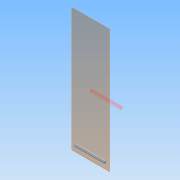
# Autodesk Inventor part: TopBottomBorder
Saved by Autodesk Inventor 2013 (Build 170138000, 138)
## iProperties
Created: 2018-07-18
Part Number: TopBottomBorder
Material: Generic
Document SubType Name: Modeling
Designer: Jeff Vyduna
Density: 1 g/cm^3
Author: Jeff Vyduna
Autodesk Inventor part; units mm, degrees
ref_plane "YZ Plane" through (0, 0, 0) normal (1, 0, 0) x (0, 1, 0)
ref_plane "XZ Plane" through (0, 0, 0) normal (0, 1, 0) x (-1, 0, 0)
ref_plane "XY Plane" through (0, 0, 0) normal (0, 0, 1) x (1, 0, 0)
ref_plane "Work Plane1" through (0, 0, 0) normal (0, 0, 1) x (1, 0, 0)
sketch "Sketch1" plane through (0, 0, 0) normal (0, 0, 1) x (1, 0, 0)
  line L0 (-264.3187, -990.6) -> (264.3188, -990.6)
  line L1 (264.3188, -990.6) -> (264.3188, -952.5)
  line L2 (264.3188, -952.5) -> (-264.3187, -952.5)
  line L3 (-264.3187, -952.5) -> (-264.3187, -990.6)
  point P0 (0, 0)
  dimension "d0" = 528.6375
  dimension "d1" = 38.1
  constraints: 8 end point, 2 parallel, 1 coincident, 1 horizontal, 1 perpendicular, 1 other
  measures "d0" distance of L1.end L2.end
  measures "d1" distance of L2.end L0.start
extrude "Extrusion1" add sketch "Sketch1" along normal blind 25.4
sketch "Sketch2" plane through (0, 0, 25.4) normal (0, 0, 1) x (1, 0, 0)
  line L0 (264.3188, -990.6) -> (264.3188, -952.5) projected
  line L1 (-264.3187, -952.5) -> (264.3188, -952.5)
  line L2 (264.3188, -952.5) -> (264.3188, -965.2)
  line L3 (264.3188, -965.2) -> (-264.3187, -965.2)
  line L4 (-264.3187, -965.2) -> (-264.3187, -952.5)
  point P0 (0, 0)
  dimension "d4" = 12.7
  constraints: 8 end point, 2 parallel, 1 horizontal, 1 perpendicular, 1 point on line
  measures "d4" distance of L1.end L2.end
extrude "Extrusion2" cut sketch "Sketch2" against normal blind 8.4646
body "Solid1"
